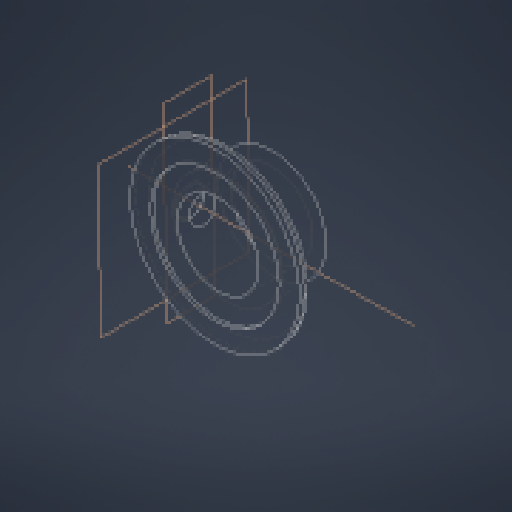
# Autodesk Inventor part: tarcza sprzęgła
Saved by Autodesk Inventor 2026.1 (Build 301233020, 233B)
## iProperties
Created: 2026-02-27
Part Number: tarcza sprzęgła
Material: Generic
Document SubType Name: Modeling
Designer: Jan
Density: 1 g/cm^3
Appearance: Default
Author: Jan
Autodesk Inventor part; units mm, degrees
ref_plane "YZ Plane" through (0, 0, 0) normal (1, 0, 0) x (0, 1, 0)
ref_plane "XZ Plane" through (0, 0, 0) normal (0, 1, 0) x (-1, 0, 0)
ref_plane "XY Plane" through (0, 0, 0) normal (0, 0, 1) x (1, 0, 0)
sketch "Sketch1" plane through (0, 0, 0) normal (1, 0, 0) x (0, 1, 0)
  line L0 (6, 3) -> (6, -3)
  line L1 (8, 1.7) -> (11.5, 1.7)
  line L2 (12.5, 2.7) -> (12.5, 3.5)
  line L3 (12.5, 2.7) -> (11.5, 2.7) construction
  line L4 (11.5, 2.7) -> (11.5, 1.7) construction
  arc A0 (11.5, 1.7) -> (12.5, 2.7) centre (11.5, 2.7) ccw
  line L5 (6, 3) -> (9.5, 3)
  line L6 (12.5, 3.5) -> (9.5, 3.5)
  line L7 (9.5, 3.5) -> (9.5, 3)
  line L8 (0, 0) -> (0, 11.4482) construction
  line L9 (8, -3) -> (8, 1.7)
  line L10 (6, -3) -> (6, -5)
  line L11 (6, -5) -> (8, -5)
  line L12 (8, -5) -> (8, -3)
  point P0 (7, 0.2)
  dimension "d0" = 6
  dimension "d1" = 3
  dimension "d5" = 0.8
  dimension "d6" = 1
  dimension "d7" = 1
  dimension "d8" = 3
  dimension "d10" = 6
  dimension "d12" = 0.5
  dimension "d14" = 3.5
  dimension "d27" = 2
  constraints: 26 end point, 5 perpendicular, 5 vertical, 2 horizontal, 2 point on circle, 1 centre point, 1 parallel, 1 tangent
  measures "d0" distance of L0.start L0.end
  measures "d1" vertical distance of L8.start L0.start
  measures "d5" distance of L2.start L2.end
  measures "d6" distance of L2.start L3.end
  measures "d7" distance of L3.end L1.end
  measures "d8" distance of L2.end L6.end
  measures "d10" distance from line of L0 L8.start
  measures "d12" distance of L6.end L5.end
  measures "d14" distance of L0.start L5.end
  measures "d27" distance of L0.end L10.end
revolve "Revolution1" add sketch "Sketch1" angle 360 about axis through (0, 0, 0) along (0, 0, 1)
ref_plane "Work Plane2" through (-7.9989, -0.1297, -1.65) normal (-0.9998686, -0.0162116, 0) x (0, 0, 1)
ref_plane "Work Plane1" through (21.3966, -11.9547, -30.348) normal (-0.9998686, -0.0162116, 0) x (0, 0, 1)
sketch "Sketch2" plane through (-7.9989, -0.1297, -1.65) normal (-0.9998686, -0.0162116, 0) x (0, 0, 1)
  circle A0 centre (1, 0) radius 1.5
  line L0 (3.35, -11.5) -> (3.35, 11.5) projected
  point P0 (1.65, 0)
  dimension "d15" = 3
  dimension "d26" = 2.35
  constraints: 1 centre point
  measures "d15" diameter of A0
  measures "d26" distance from line of L0 A0.centre
hole "Hole1" at (-7.9989, -0.1297, -0.65) direction (0.9998686, 0.0162116, 0) diameter 4 depth 8.8 tip angle 118
chamfer "Chamfer1" distance 0.2 angle 45 2 edges at (-7.7796, 1.8651, -0.8399) (-7.7125, -2.1253, -0.6469)
ref_plane "Work Plane4" through (-7.9989, -0.1297, 1.55) normal (-0.9998686, -0.0162116, 0) x (0.0162116, -0.9998686, 0)
equation "\"d1\" = 0.5 * d0"
equation "\"d7\" = d6"
body "Solid1"
